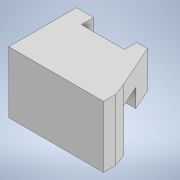
# Autodesk Inventor part: Część1
Saved by Autodesk Inventor 2021 (Build 250183000, 183)
## iProperties
Created: 2024-04-13
Part Number: Część1
Material: Ogólny
Document SubType Name: Modeling
Designer: Dawidek
Density: 1 g/cm^3
Appearance: Domyślna
Author: Dawidek
Autodesk Inventor part; units mm, degrees
ref_plane "YZ Plane" through (0, 0, 0) normal (1, 0, 0) x (0, 1, 0)
ref_plane "XZ Plane" through (0, 0, 0) normal (0, 1, 0) x (-1, 0, 0)
ref_plane "XY Plane" through (0, 0, 0) normal (0, 0, 1) x (1, 0, 0)
sketch "Szkic1" plane through (0, 0, 0) normal (0, 0, 1) x (1, 0, 0)
  line L0 (0, 0) -> (77, 0)
  line L1 (77, 0) -> (77, 50)
  line L2 (77, 50) -> (0, 50)
  line L3 (0, 50) -> (0, 0)
  dimension "d0" = 77
  dimension "d1" = 50
  constraints: 8 end point, 3 perpendicular, 1 horizontal
  measures "d0" distance of L0.start L0.end
  measures "d1" distance of L0.end L1.end
extrude "Wyciągnięcie proste1" add sketch "Szkic1" along normal blind 10
sketch "Szkic2" plane through (0, 0, 0) normal (0, -1, 0) x (1, 0, 0)
  line L0 (77, 0) -> (0, 0) projected
  line L1 (0, 0) -> (77, 0)
  line L2 (77, 0) -> (0, 0)
  line L3 (0, 0) -> (0, -10)
  line L4 (0, -10) -> (73.2222, -10)
  line L5 (77, 0) -> (0, 0)
  line L6 (73.2222, -10) -> (77, 0)
  dimension "d6" = 10
  constraints: 12 end point, 2 collinear, 1 horizontal, 1 perpendicular
  measures "d6" distance of L0.end L3.end
extrude "Wyciągnięcie proste2" add sketch "Szkic2" against normal blind 50
sketch "Szkic3" plane through (0, 50, 10) normal (0, 1, 0) x (1, 0, 0)
  line L0 (0, 20) -> (0, 0) projected
  line L1 (0, 20) -> (0, 38)
  line L2 (77, 10) -> (73.2222, 20) projected
  line L3 (73.2222, 20) -> (66.4222, 38)
  line L4 (66.4222, 38) -> (0, 38)
  point P0 (0, 10)
  dimension "d9" = 18
  constraints: 6 end point, 1 collinear, 1 horizontal, 1 vertical
  measures "d9" distance of L0.start L1.end
sketch "Szkic4" plane through (0, 50, 10) normal (0, 1, 0) x (1, 0, 0)
  line L0 (0, 20) -> (0, 0) projected
  line L1 (0, 20) -> (0, 38)
  line L2 (73.2222, 20) -> (0, 20) projected
  line L3 (0, 20) -> (73.2222, 20)
  line L4 (73.2222, 20) -> (65.2222, 38)
  line L5 (65.2222, 38) -> (0, 38)
  point P0 (0, 10)
  dimension "d10" = 18
  constraints: 8 end point, 1 collinear, 1 parallel, 1 vertical
  measures "d10" distance of L0.start L1.end
extrude "Wyciągnięcie proste3" add sketch "Szkic4" against normal blind 15
sketch "Szkic5" plane through (0, 50, 10) normal (0, 1, 0) x (1, 0, 0)
  line L0 (0, 38) -> (65.2222, 38) projected
  line L1 (0, 38) -> (0, 55)
  line L2 (0, 38) -> (65.2222, 38)
  line L3 (65.2222, 38) -> (73.2222, 20) projected
  line L4 (57.6666, 55) -> (65.2222, 38)
  line L5 (0, 55) -> (14, 55)
  line L6 (14, 55) -> (14, 45)
  line L7 (14, 45) -> (49, 45)
  line L8 (49, 45) -> (49, 55)
  line L9 (49, 55) -> (57.6666, 55)
  point P0 (0, 10)
  dimension "d13" = 17
  dimension "d14" = 14
  dimension "d15" = 10
  dimension "d16" = 35
  constraints: 16 end point, 3 perpendicular, 3 point on line, 2 collinear, 1 horizontal, 1 vertical
  measures "d13" distance of L0.start L1.end
  measures "d14" distance of L1.end L5.end
  measures "d15" distance of L5.end L6.end
  measures "d16" distance of L6.end L7.end
extrude "Wyciągnięcie proste4" add sketch "Szkic5" against normal blind 30
